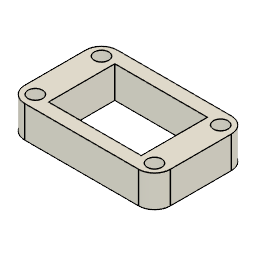
Neck (Autodesk Fusion 360 design; units mm, degrees)
part number: 2026-07-06-11-28-03-272
Autodesk Fusion 360 part; units mm, degrees
sketch "Sketch1" plane through (0, 0, 0) normal (0, 1, 0) x (1, 0, 0)
  line L0 (0, 0) -> (35, 0)
  line L1 (35, 0) -> (35, 25)
  line L2 (35, 25) -> (0, 25)
  line L3 (0, 25) -> (0, 0)
  line L4 (-10, 30) -> (45, 30)
  line L5 (45, 30) -> (45, -5)
  line L6 (45, -5) -> (-10, -5)
  line L7 (-10, -5) -> (-10, 30)
  circle A0 centre (-5, 0) radius 2.75
  circle A1 centre (-5, 25) radius 2.75
  circle A2 centre (40, 0) radius 2.75
  circle A3 centre (40, 25) radius 2.75
  dimension "d1" = 35
  dimension "d2" = 25
  dimension "d3" = 55
  dimension "d4" = 35
  dimension "d5" = 5
  dimension "d6" = 10
  dimension "d7" = 5.5
  dimension "d8" = 5
  dimension "d9" = 5
  dimension "d10" = 5.5
  dimension "d11" = 5
  dimension "d12" = 5
  dimension "d13" = 5.5
  dimension "d14" = 5
  dimension "d15" = 5
  dimension "d16" = 5.5
  dimension "d17" = 5
  dimension "d18" = 5
  constraint horizontal L0
  constraint vertical L1
  constraint horizontal L2
  constraint vertical L3
  constraint coincident L0.start L3.end
  constraint horizontal L4
  constraint vertical L5
  constraint horizontal L6
  constraint vertical L7
  measures "d1" distance of L0.start L0.end
  measures "d2" distance of L0.start L2.end
  measures "d3" distance of L4.start L4.end
  measures "d4" distance of L4.start L6.end
  measures "d5" distance of L0 L6
  measures "d6" distance of L3 L7
  measures "d7" diameter of A0
  measures "d8" distance of L6 A0.centre
  measures "d9" distance of L7 A0.centre
  measures "d10" diameter of A1
  measures "d11" distance of L7 A1.centre
  measures "d12" distance of L4 A1.centre
  measures "d13" diameter of A2
  measures "d14" distance of L5 A2.centre
  measures "d15" distance of L6 A2.centre
  measures "d16" diameter of A3
  measures "d17" distance of L5 A3.centre
  measures "d18" distance of L4 A3.centre
extrude "Extrude1" add sketch "Sketch1" along normal blind 12 contours L4 L5 L6 L7 | A0 | A1 | A2 | A3
extrude "Extrude2" cut sketch "Sketch1" along normal blind 4.5 contours A0 | A1 | A2 | A3
ref_plane "WorkPlane1" through (0, 12, 0) normal (0, 1, 0) x (0, 0, 1)
sketch "Sketch2" plane through (0, 12, 0) normal (0, 1, 0) x (1, 0, 0)
  circle A0 centre (-5, 25) radius 2.75
  circle A1 centre (40, 0) radius 2.75
  circle A2 centre (40, 25) radius 2.75
  circle A3 centre (-5, 0) radius 2.75
  circle A4 centre (-5, 0) radius 1.7
  circle A5 centre (-5, 25) radius 1.7
  circle A6 centre (40, 25) radius 1.7
  circle A7 centre (40, 0) radius 1.7
  dimension "d24" = 5.5
  dimension "d26" = 5.5
  dimension "d28" = 5.5
  dimension "d29" = 5.5
  dimension "d32" = 3.4
  dimension "d33" = 3.4
  dimension "d34" = 3.4
  dimension "d35" = 3.4
  constraint concentric A3 A4
  constraint concentric A0 A5
  constraint concentric A2 A6
  constraint concentric A1 A7
  measures "d24" diameter of A0
  measures "d26" diameter of A1
  measures "d28" diameter of A2
  measures "d29" diameter of A3
  measures "d32" diameter of A4
  measures "d33" diameter of A5
  measures "d34" diameter of A6
  measures "d35" diameter of A7
extrude "Extrude3" cut sketch "Sketch2" against normal blind 4.5 contours A0 | A1 | A2 | A3 | A4 | A5 | A6 | A7
extrude "Extrude4" cut sketch "Sketch2" against normal blind 20 contours A4 | A5 | A6 | A7
fillet "Fillet1" radius 6 4 edges at (45, 6, -30) (45, 6, 5) (-10, 6, 5) (-10, 6, -30)
